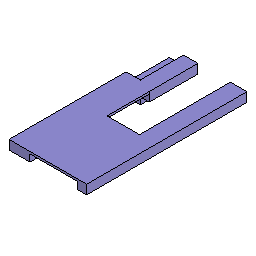
Capac Arc Dreapta (Autodesk Fusion 360 design; units mm, degrees)
part number: 2026-06-02-22-17-47-582
Autodesk Fusion 360 part; units mm, degrees
sketch "Sketch1" plane through (0, 0, 0) normal (0, 0, 1) x (1, 0, 0)
  line L0 (16.1782, -61.5942) -> (11.8447, -61.5942)
  line L1 (16.1782, -34.0942) -> (16.1782, -52.4272)
  line L2 (11.8447, -61.5942) -> (11.8447, -124.5942)
  line L3 (0, -124.5942) -> (11.8447, -124.5942)
  line L4 (0, -58.5) -> (0, -124.5942)
  line L5 (0, -55) -> (0, -58.5)
  line L6 (16.1782, -34.0942) -> (0, -34.0942)
  line L7 (34.5112, -52.4272) -> (34.5112, -34.0942)
  line L8 (34.5112, -34.0942) -> (43.8447, -34.0942)
  line L9 (43.8447, -124.5942) -> (43.8447, 39.5803)
  line L10 (38.8447, -124.5942) -> (43.8447, -124.5942)
  line L11 (38.8447, -121.5942) -> (38.8447, -124.5942)
  line L12 (38.8447, -124.5942) -> (38.8447, -61.5942)
  line L13 (38.8447, -61.5942) -> (34.5112, -61.5942)
  line L14 (36.4949, -85.428) -> (14.1949, -85.428)
  line L15 (35.8447, -61.5942) -> (35.8447, -124.5942)
  line L16 (35.8447, -124.5942) -> (14.1949, -124.5942)
  line L17 (14.1949, -124.5942) -> (14.1949, -61.5942)
  line L18 (16.1782, -52.4272) -> (16.1782, -61.5942)
  line L19 (0, -55) -> (0, -34.0942)
  line L20 (34.5112, -52.4272) -> (34.5112, -61.5942)
  line L21 (11.8447, -124.5942) -> (14.1949, -124.5942)
  line L22 (35.8447, -124.5942) -> (38.8447, -124.5942)
  circle A0 centre (3.5, -37.5942) radius 3.5
  circle A1 centre (3.5, -37.5942) radius 2
  line L23 (34.5112, -61.5942) -> (34.5112, -85.428)
  line L24 (16.1782, -61.5942) -> (16.1782, -85.428)
  line L25 (0, -58.5) -> (8, -58.5)
  line L26 (8, -58.5) -> (8, -34.0942)
  line L27 (0, -60.5) -> (10, -60.5)
  line L28 (10, -60.5) -> (10, -34.0942)
  point P0 (0, -58.5)
  point P1 (0, -34.0942)
  dimension "d522" = 51.3338
  dimension "d523" = 14.1949
  dimension "d524" = 36.4949
  dimension "d525" = 43.8447
  dimension "d526" = 11.8447
  dimension "d527" = 16.1782
  dimension "d528" = 34.0942
  dimension "d529" = 34.5112
  dimension "d530" = 35.8447
  dimension "d531" = 38.8447
  dimension "d532" = 4.3335
  dimension "d533" = 164.1745
  dimension "d534" = 63
  dimension "d535" = 90.5
  dimension "d536" = 87.5
  dimension "d537" = 27.5
  dimension "d538" = 23.8338
  dimension "d539" = 21.6498
  dimension "d540" = 66.0942
  dimension "d541" = 20.9058
  dimension "d542" = 18.333
  dimension "d546" = 3.5
  dimension "d547" = 4
  dimension "d570" = 24.4058
  dimension "d571" = 8
  dimension "d576" = 2
  constraint perpendicular L0 L18
  constraint perpendicular L6 L19
  constraint perpendicular L13 L20
  constraint perpendicular L17 L21
  constraint perpendicular L11 L22
  constraint vertical origin P1
  constraint perpendicular L1 L6
  constraint parallel L6 L10
  constraint collinear L6 L8
  constraint collinear L5 L19
  constraint vertical origin L3.start
  constraint collinear L1 L18
  constraint equal L1 L7
  constraint perpendicular L9 L10
  constraint perpendicular L10 L11
  constraint perpendicular L10 L12
  constraint collinear L3 L10
  constraint collinear L10 L16
  constraint perpendicular L7 L8
  constraint coincident L14.end L17
  constraint coincident L8.end L9
  constraint equal L2 L17
  constraint tangent L6 A0
  constraint tangent L19 A0
  constraint concentric A0 A1
  constraint coincident L14 L23.end
  constraint perpendicular L14 L23
  constraint coincident L14 L24.end
  constraint perpendicular L14 L24
  constraint coincident P0 L4.start
  constraint perpendicular L4 L25
  constraint coincident L6 L26.end
  constraint perpendicular L6 L26
  measures "d522" distance of L6 L14
  measures "d523" distance of L14.end L19
  measures "d524" distance of L14.start L19
  measures "d525" distance of origin L9
  measures "d526" distance of origin L2
  measures "d527" distance of origin L1
  measures "d528" distance of origin L8
  measures "d529" distance of origin L7
  measures "d530" distance of origin L15
  measures "d531" distance of origin L12
  measures "d532" distance of L1 L2
  measures "d533" distance of L9.end L10
  measures "d534" distance of L10 L13
  measures "d535" distance of L8 L10
  measures "d536" distance of L8 L11.start
  measures "d537" distance of L8 L15.start
  measures "d538" distance of L0 L14
  measures "d539" distance of L14.end L15
  measures "d540" distance of P0 L10
  measures "d541" distance of L5.start L8
  measures "d542" distance of L7.start L8
  measures "d546" radius of A0
  measures "d547" diameter of A1
  measures "d570" distance of P0 P1
  measures "d571" distance of P0 L25.end
extrude "Extrude1" add sketch "Sketch1" along normal blind 5.2 contours L0 L1 L2 L3 L4 L6 L18 L27 L28 | L4 L6 L25 L26 L27 L28 | L7 L8 L9 L10 L11 L12 L13 L20 | L5 L6 L19 A0 L25 L26 | L6 L19 A0 | A0 | A1 makes body 1 at (39.0669, -43.2609, 0) makes body 2 at (9.341, -43.2609, 0)
extrude "Extrude2" add sketch "Sketch1" along normal blind 1.2 from surface at 4 contours L0 L2 L17 L21 | L14 L15 L16 L17 | L11 L12 L13 L15 L22 bodies 1 2
extrude "Extrude3" add sketch "Sketch1" against normal blind 7 contours A0 bodies 1
extrude "Extrude4" cut sketch "Sketch1" along normal blind 2 contours A1 bodies 1
extrude "Extrude7" add sketch "Sketch1" against normal blind 5 contours L4 L6 L25 L26 L27 L28 | L5 L6 L19 A0 L25 L26 | L6 L19 A0 | A1 bodies 1
extrude "Extrude8" cut sketch "Sketch1" along normal blind 6 contours L5 L6 L19 A0 L25 L26 | L6 L19 A0 | A0 | A1 bodies 1
extrude "Extrude9" cut 1 faces at (3.7436, -38.2148, -5) along direction (0, 0, 1) blind 3 on bodies 1 bodies 1
move_body "Move1" bodies 1 to x (1, 0, 0) y (0, 1, 0) z (0, 0, 1) at (0, 0, 53)
extrude "Extrude5" add 1 faces at (14.1949, -77.4834, 57.4) along direction (1, 0, 0) blind 2 on bodies 1 bodies 1
extrude "Extrude6" add 1 faces at (35.8447, -69.5388, 57.4) along direction (-1, 0, 0) up to surface (1.3335 mm away) on bodies 1 bodies 1
equation "d550 = --2 mm"
